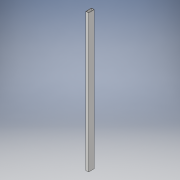
# Autodesk Inventor part: main beam
Saved by Autodesk Inventor 2017 (Build 210142000, 142)
## iProperties
Created: 2017-12-26
Part Number: main beam
Material: Generic
Document SubType Name: Modeling
Designer: Micah
Density: 1 g/cm^3
Appearance: Default
Author: Micah
Autodesk Inventor part; units mm, degrees
ref_plane "YZ Plane" through (0, 0, 0) normal (1, 0, 0) x (0, 1, 0)
ref_plane "XZ Plane" through (0, 0, 0) normal (0, 1, 0) x (-1, 0, 0)
ref_plane "XY Plane" through (0, 0, 0) normal (0, 0, 1) x (1, 0, 0)
sketch "Sketch2" plane through (0, 0, 0) normal (0, 1, 0) x (-1, 0, 0)
  line L0 (0, 0) -> (-25.4, 0)
  line L1 (-25.4, 0) -> (0, 0)
  line L2 (0, 0) -> (0, -50.8)
  line L3 (0, -50.8) -> (-25.4, -50.8)
  line L4 (-25.4, -50.8) -> (-25.4, 0)
  line L5 (-22.225, -47.625) -> (-3.175, -47.625)
  line L6 (-3.175, -47.625) -> (-3.175, -3.175)
  line L7 (-3.175, -3.175) -> (-22.225, -3.175)
  line L8 (-22.225, -3.175) -> (-22.225, -47.625)
  dimension "d2" = 25.4
  dimension "d3" = 50.8
  dimension "d4" = 19.05
  dimension "d5" = 44.45
  dimension "d6" = 3.175
  dimension "d7" = 3.175
  constraints: 18 end point, 4 parallel, 2 horizontal, 2 perpendicular
  measures "d2" distance of L2.end L3.end
  measures "d3" distance of L1.end L2.end
  measures "d4" distance of L7.end L6.end
  measures "d5" distance of L6.end L5.end
  measures "d6" distance between parallel lines of L4 L8
  measures "d7" distance between parallel lines of L5 L3
extrude "Extrusion1" add sketch "Sketch2" along normal blind 1219.2
body "Solid1"
